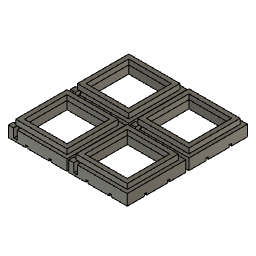
Bitleaf (Autodesk Fusion 360 design; units mm, degrees)
Autodesk Fusion 360 part; units mm, degrees
note: some values were not read from the file. Chosen so that the rebuilt part matches the saved one: which bodies a step acts on; which face or edge a step refers to. Set by a fixed rule: which sketch regions a step uses.
sketch "Skizze1" plane through (0, 0, 0) normal (0, 0, 1) x (1, 0, 0)
  line L0 (0, 0) -> (66.6, 0)
  line L1 (66.6, 0) -> (66.6, -66.6)
  line L2 (66.6, -66.6) -> (0, -66.6)
  line L3 (0, -66.6) -> (0, 0)
  dimension "d1" = 66.6
  dimension "d2" = 66.6
  constraint horizontal L0
  constraint vertical L1
  constraint horizontal L2
  constraint vertical L3
  constraint coincident L0.start L3.end
  measures "d1" distance of L0.start L0.end
  measures "d2" distance of L0.start L2.end
extrude "Extrusion1" add sketch "Skizze1" along normal blind 20 makes body 1
shell "Schale1" thickness 7 outward yes removed faces 1 at (22.2, -22.2, 20) on bodies 1
sketch "Skizze2" plane through (0, 0, 0) normal (0, 0, 1) x (-1, 0, 0)
  line L0 (0, 66.6) -> (-66.6, 66.6)
  line L1 (-66.6, 66.6) -> (-66.6, 0)
  line L2 (-66.6, 0) -> (0, 0)
  line L3 (0, 0) -> (0, 66.6)
  line L4 (0, 0) -> (-66.6, 0)
  line L5 (-66.6, 0) -> (-66.6, 4)
  line L6 (-66.6, 4) -> (0, 4)
  line L7 (0, 4) -> (0, 0)
  line L8 (0, 0) -> (-4, 0)
  line L9 (-4, 0) -> (-4, 66.6)
  line L10 (-4, 66.6) -> (0, 66.6)
  line L11 (0, 66.6) -> (0, 0)
  line L12 (0, 66.6) -> (-66.6, 66.6)
  line L13 (-66.6, 66.6) -> (-66.6, 62.6)
  line L14 (-66.6, 62.6) -> (0, 62.6)
  line L15 (0, 62.6) -> (0, 66.6)
  line L16 (-66.6, 0) -> (-62.6, 0)
  line L17 (-62.6, 0) -> (-62.6, 66.6)
  line L18 (-62.6, 66.6) -> (-66.6, 66.6)
  line L19 (-66.6, 66.6) -> (-66.6, 0)
  dimension "d6" = 66.6
  dimension "d7" = 4
  dimension "d8" = 4
  dimension "d9" = 66.6
  dimension "d10" = 66.6
  dimension "d11" = 4
  dimension "d12" = 4
  dimension "d13" = 66.6
  constraint horizontal L4
  constraint vertical L5
  constraint horizontal L6
  constraint vertical L7
  constraint coincident L2.end L3.start
  constraint horizontal L8
  constraint vertical L9
  constraint horizontal L10
  constraint vertical L11
  constraint horizontal L12
  constraint vertical L13
  constraint horizontal L14
  constraint vertical L15
  constraint coincident L0.start L3.end
  constraint horizontal L16
  constraint vertical L17
  constraint horizontal L18
  constraint vertical L19
  constraint coincident L1.end L2.start
  measures "d6" distance of L2.end L1.end
  measures "d7" distance of L2.end L6.end
  measures "d8" distance of L2.end L8.end
  measures "d9" distance of L2.end L0.start
  measures "d10" distance of L0.start L0.end
  measures "d11" distance of L0.start L14.end
  measures "d12" distance of L1.end L16.end
  measures "d13" distance of L1.end L0.end
extrude "Extrusion2" cut sketch "Skizze2" against normal blind 42 contours L6 L9 L14 L17 bodies 1
sketch "Skizze3" plane through (0, 0, 0) normal (0, 1, 0) x (1, 0, 0)
  line L0 (-7, 7) -> (-2, 7)
  line L1 (-2, 7) -> (-2, 2)
  line L2 (-2, 2) -> (-7, 2)
  line L3 (-7, 2) -> (-7, 7)
  dimension "d16" = 5
  dimension "d17" = 5
  constraint horizontal L0
  constraint vertical L1
  constraint horizontal L2
  constraint vertical L3
  measures "d16" distance of L0.start L0.end
  measures "d17" distance of L0.start L2.end
sketch "Skizze4" plane through (0, -73.6, 0) normal (0, -1, 0) x (1, 0, 0)
  line L0 (-7, -7) -> (73.6, -7)
  line L1 (73.6, -7) -> (73.6, 20)
  line L2 (73.6, 20) -> (-7, 20)
  line L3 (-7, 20) -> (-7, -7)
  line L4 (-7, -7) -> (-2, -7)
  line L5 (-2, -7) -> (-2, -2)
  line L6 (-2, -2) -> (-7, -2)
  line L7 (-7, -2) -> (-7, -7)
  line L8 (73.6, -7) -> (68.6, -7)
  line L9 (68.6, -7) -> (68.6, -2)
  line L10 (68.6, -2) -> (73.6, -2)
  line L11 (73.6, -2) -> (73.6, -7)
  dimension "d18" = 5
  dimension "d19" = 5
  dimension "d20" = 5
  dimension "d21" = 5
  constraint horizontal L4
  constraint vertical L5
  constraint horizontal L6
  constraint vertical L7
  constraint coincident L0.start L3.end
  constraint horizontal L8
  constraint vertical L9
  constraint horizontal L10
  constraint vertical L11
  constraint coincident L0.end L1.start
  measures "d18" distance of L0.start L4.end
  measures "d19" distance of L0.start L6.end
  measures "d20" distance of L0.end L8.end
  measures "d21" distance of L0.end L10.end
extrude "Extrusion3" cut sketch "Skizze4" against normal blind 570 contours L0 L3 L4 L5 L6 L7 bodies 1
sketch "Skizze5" plane through (0, -73.6, 0) normal (0, -1, 0) x (1, 0, 0)
  line L0 (-2, -2) -> (-2, -7)
  line L1 (-2, -7) -> (73.6, -7)
  line L2 (73.6, -7) -> (73.6, 20)
  line L3 (73.6, 20) -> (-7, 20)
  line L4 (-7, 20) -> (-7, -2)
  line L5 (-7, -2) -> (-2, -2)
  line L6 (73.6, -7) -> (68.6, -7)
  line L7 (68.6, -7) -> (68.6, -2)
  line L8 (68.6, -2) -> (73.6, -2)
  line L9 (73.6, -2) -> (73.6, -7)
  dimension "d24" = 5
  dimension "d25" = 5
  constraint horizontal L6
  constraint vertical L7
  constraint horizontal L8
  constraint vertical L9
  constraint coincident L1.end L2.start
  measures "d24" distance of L1.end L6.end
  measures "d25" distance of L1.end L8.end
extrude "Extrusion4" cut sketch "Skizze5" against normal blind 280 contours L1 L2 L6 L7 L8 L9 bodies 1
sketch "Skizze6" plane through (68.6, 0, 0) normal (1, 0, 0) x (0, 1, 0)
  line L0 (7, -7) -> (7, -2)
  line L1 (7, -2) -> (-73.6, -2)
  line L2 (-73.6, -2) -> (-73.6, -7)
  line L3 (-73.6, -7) -> (7, -7)
  line L4 (7, -7) -> (2, -7)
  line L5 (2, -7) -> (2, -2)
  line L6 (2, -2) -> (7, -2)
  line L7 (7, -2) -> (7, -7)
  dimension "d28" = 5
  dimension "d29" = 5
  constraint horizontal L4
  constraint vertical L5
  constraint horizontal L6
  constraint vertical L7
  constraint coincident L0.start L3.end
  measures "d28" distance of L0.start L4.end
  measures "d29" distance of L0.start L0.end
extrude "Extrusion5" cut sketch "Skizze6" against normal blind 135 contours L0 L1 L3 L4 L5 L6 L7 bodies 1
sketch "Skizze7" plane through (68.6, 0, 0) normal (1, 0, 0) x (0, 1, 0)
  line L0 (2, -7) -> (2, -2)
  line L1 (2, -2) -> (-73.6, -2)
  line L2 (-73.6, -2) -> (-73.6, -7)
  line L3 (-73.6, -7) -> (2, -7)
  line L4 (-73.6, -7) -> (-68.6, -7)
  line L5 (-68.6, -7) -> (-68.6, -2)
  line L6 (-68.6, -2) -> (-73.6, -2)
  line L7 (-73.6, -2) -> (-73.6, -7)
  dimension "d32" = 5
  dimension "d33" = 5
  constraint horizontal L4
  constraint vertical L5
  constraint horizontal L6
  constraint vertical L7
  constraint coincident L2.end L3.start
  measures "d32" distance of L2.end L4.end
  measures "d33" distance of L2.end L1.end
extrude "Extrusion6" cut sketch "Skizze7" against normal blind 145 contours L1 L2 L3 L4 L5 L6 L7 bodies 1
sketch "Skizze8" plane through (0, -66.6, 0) normal (0, 1, 0) x (-1, 0, 0)
  line L0 (-66.6, 0) -> (0, 0)
  line L1 (0, 0) -> (0, 20)
  line L2 (0, 20) -> (-66.6, 20)
  line L3 (-66.6, 20) -> (-66.6, 0)
  line L4 (-66.6, 0) -> (-61.6, 0)
  line L5 (-61.6, 0) -> (-61.6, 16)
  line L6 (-61.6, 16) -> (-66.6, 16)
  line L7 (-66.6, 16) -> (-66.6, 0)
  dimension "d36" = 5
  dimension "d37" = 16
  constraint horizontal L4
  constraint vertical L5
  constraint horizontal L6
  constraint vertical L7
  constraint coincident L0.start L3.end
  measures "d36" distance of L0.start L4.end
  measures "d37" distance of L0.start L6.end
extrude "Extrusion7" cut sketch "Skizze8" against normal blind 20 contours L0 L3 L4 L5 L6 L7 bodies 1
sketch "Skizze9" plane through (66.6, 0, 0) normal (-1, 0, 0) x (0, -1, 0)
  line L0 (0, 0) -> (73.6, 0)
  line L1 (73.6, 0) -> (73.6, 16)
  line L2 (73.6, 16) -> (66.6, 16)
  line L3 (66.6, 16) -> (66.6, 20)
  line L4 (66.6, 20) -> (0, 20)
  line L5 (0, 20) -> (0, 0)
  line L6 (66.6, 16) -> (61.6, 16)
  line L7 (61.6, 16) -> (61.6, 0)
  line L8 (61.6, 0) -> (66.6, 0)
  line L9 (66.6, 0) -> (66.6, 16)
  dimension "d40" = 5
  constraint horizontal L6
  constraint vertical L7
  constraint horizontal L8
  constraint vertical L9
  constraint coincident L2.end L3.start
  measures "d40" distance of L2.end L6.end
extrude "Extrusion8" cut sketch "Skizze9" against normal blind 19 contours L0 L6 L7 L8 L9 bodies 1
sketch "Skizze10" plane through (0, 0, 0) normal (0, 0, 1) x (1, 0, 0)
  circle A0 centre (-80, 15) radius 1.5
  line L0 (-78.8067, 15.9088) -> (-74.8067, 15.9088)
  line L1 (-74.8067, 15.9088) -> (-74.8067, 14.0729)
  line L2 (-74.8067, 14.0729) -> (-78.8067, 14.0729)
  line L3 (-78.8067, 14.0729) -> (-78.8067, 15.9088)
  dimension "d43" = 3
  dimension "d44" = 4
  dimension "d45" = 1.836
  constraint horizontal L0
  constraint vertical L1
  constraint horizontal L2
  constraint vertical L3
  constraint coincident A0 L0.start
  measures "d43" diameter of A0
  measures "d44" distance of L0.start L0.end
  measures "d45" distance of L0.start L2.end
sketch "Skizze11" plane through (0, 0, 0) normal (0, 0, 1) x (1, 0, 0)
sketch "Skizze12" plane through (0, 0, 0) normal (0, 0, 1) x (1, 0, 0)
  line L0 (-74.8, 15) -> (-73.607, 15)
  circle A0 centre (-73.607, 15) radius 1.5
  dimension "d46" = 1.193
  dimension "d47" = 3
  constraint horizontal L0
  constraint coincident L0.end A0.centre
  measures "d46" distance of L0.start L0.end
  measures "d47" diameter of A0
extrude "Extrusion9" add sketch "Skizze10" sketch "Skizze12" along normal blind 3 separate body of sketch 2 makes body 2
move_body "Verschieben1" bodies 2 to x (1, 0, 0) y (0, 1, 0) z (0, 0, 1) at (60, -70, 0)
extrude "Extrusion10" add 2 faces at (71.2667, -63.2667, 16) (63.2667, -68.9333, 16) along direction (0, 0, -1) blind 4 on bodies 1 bodies 1
extrude "Extrusion11" cut 1 faces at (44.4, -71.2667, 20) along direction (0, 0, -1) blind 5 on bodies 1 bodies 1
move_body "Verschieben2" bodies 2 to x (1, 0, 0) y (0, 1, 0) z (0, 0, 1) at (9, 0, 17)
move_body "Verschieben3" bodies 2 to x (1, 0, 0) y (0, 1, 0) z (0, 0, 1) at (-2.1624, 3.0539, -2.6132)
sketch "Skizze13" plane through (0, 0, 15) normal (0, 0, 1) x (-1, 0, 0)
  line L0 (0, 66.6) -> (0, 0)
  line L1 (0, 0) -> (-66.6, 0)
  line L2 (-66.6, 0) -> (-66.6, 66.6)
  line L3 (-66.6, 66.6) -> (0, 66.6)
  line L4 (7, 73.6) -> (-73.6, 73.6)
  line L5 (-73.6, 73.6) -> (-73.6, -7)
  line L6 (-73.6, -7) -> (7, -7)
  line L7 (7, -7) -> (7, 73.6)
extrude "Extrusion12" add sketch "Skizze10" sketch "Skizze12" along normal blind 3 separate body of sketch 2 makes body 3
move_body "Verschieben4" bodies 2 to x (1, 0, 0) y (0, 1, 0) z (0, 0, 1) at (-9, 0, 0)
sketch "Skizze14" plane through (0, 0, 15) normal (0, 0, 1) x (-1, 0, 0)
sketch "Skizze15" plane through (0, 0, 0) normal (0, 0, 1) x (1, 0, 0)
  circle A0 centre (-44.5, -48.5) radius 1.8
  circle A1 centre (-50.5, -48.5) radius 1.8
  line L0 (-50.5, -48.5) -> (-44.5, -48.5)
  line L1 (-47.5, -47) -> (-47.5, -50)
  line L2 (-45.0171, -47) -> (-50, -47)
  line L3 (-50, -47) -> (-50, -50)
  line L4 (-50, -50) -> (-45.0171, -50)
  line L5 (-45.0171, -50) -> (-45.0171, -47)
  constraint coincident A1.centre L0.start
  constraint coincident A0.centre L0.end
  constraint horizontal L0
  constraint perpendicular L0 L1
  constraint horizontal L2
  constraint vertical L3
  constraint horizontal L4
  constraint vertical L5
extrude "Extrusion13" add sketch "Skizze15" along normal blind 3 separate body contours A0 L2 L4 L5 | A0 L0 L2 L5 | A0 L0 L1 L2 | A0 L0 L1 L4 | A0 L0 L4 L5 makes body 4
move_body "Verschieben5" bodies 2 to x (1, 0, 0) y (0, 1, 0) z (0, 0, 1) at (-7, 0, 0)
sketch "Skizze16" plane through (0, 0, 15) normal (0, 0, 1) x (-1, 0, 0)
  line L0 (7, 50) -> (-73.6, 50)
  line L1 (7, 50) -> (7, 15)
  line L2 (7, 15) -> (-73.6, 15)
  line L3 (-73.6, 15) -> (-73.6, 50)
  line L4 (-73.6, 73.6) -> (-50, 73.6)
  line L5 (-50, 73.6) -> (-15, 73.6)
  line L6 (-15, 73.6) -> (-15, -7)
  line L7 (-15, -7) -> (-50, -7)
  line L8 (-50, -7) -> (-50, 73.6)
  dimension "d60" = 23.6
  constraint horizontal L0
  constraint perpendicular L0 L1
  constraint perpendicular L1 L2
  constraint perpendicular L0 L3
  constraint horizontal L4
  constraint horizontal L5
  constraint vertical L6
  constraint horizontal L7
  constraint vertical L8
  measures "d60" distance of L4.start L4.end
copy_body "Körper kopieren/einfügen1" bodies 4 makes body 5
move_body "Verschieben6" bodies 5 to x (1, 0, 0) y (0, 1, 0) z (0, 0, 1) at (40.5, 0, 12)
move_body "Verschieben7" bodies 5 to x (1, 0, 0) y (0, 1, 0) z (0, 0, 1) at (-8, 0, 0)
sketch "Skizze17" plane through (0, 0, 0) normal (1, 0, 0) x (0, 1, 0)
sketch "Skizze18" plane through (0, 0, 0) normal (0, 0, 1) x (1, 0, 0)
move_body "Verschieben8" bodies 4 to x (1, 0, 0) y (0, 1, 0) z (0, 0, 1) at (10, 0, 0)
move_body "Verschieben9" bodies 5 to x (1, 0, 0) y (0, 1, 0) z (0, 0, 1) at (8, 0, 0)
split "Teilen1" by bodies 5 bodies 1 makes body 6 at (22.2, -71.2667, 15)
move_body "Verschieben10" bodies 5 to x (1, 0, 0) y (0, 1, 0) z (0, 0, 1) at (0, 32, 0)
split "Teilen2" by bodies 5 bodies 6 makes body 7 at (22.2, -71.2667, 15)
move_body "Verschieben11" bodies 5 to x (0, -1, 0) y (1, 0, 0) z (0, 0, 1) at (33, 0, 0)
split "Teilen3" by bodies 5 bodies 7 makes body 8 at (44.4, -71.2667, 15)
move_body "Verschieben12" bodies 5 to x (1, 0, 0) y (0, 1, 0) z (0, 0, 1) at (32, 0, 0)
split "Teilen4" by bodies 5 bodies 8 makes body 9 at (44.4, -71.2667, 15)
move_body "Verschieben13" bodies 5 to x (0, -1, 0) y (1, 0, 0) z (0, 0, 1) at (66.6, 32, 0)
split "Teilen5" by bodies 5 bodies 9 makes body 10 at (44.4, -71.2667, 15)
move_body "Verschieben14" bodies 5 to x (1, 0, 0) y (0, 1, 0) z (0, 0, 1) at (0, -32, 0)
split "Teilen6" by bodies 5 bodies 10 makes body 11 at (22.2, -71.2667, 15)
move_body "Verschieben15" bodies 5 to x (0, -1, 0) y (1, 0, 0) z (0, 0, 1) at (97, 0, 0)
split "Teilen7" by bodies 5 bodies 11 makes body 12 at (13.3333, -71.2667, 15)
move_body "Verschieben16" bodies 5 to x (1, 0, 0) y (0, 1, 0) z (0, 0, 1) at (-32, 0, 0)
split "Teilen8" by bodies 5 bodies 12 makes body 13 at (71.2667, -63.4, 15)
move_body "Verschieben17" bodies 5 to x (1, 0, 0) y (0, 1, 0) z (0, 0, 1) at (0, -30, 0)
move_body "Verschieben18" bodies 2 to x (1, 0, 0) y (0, 1, 0) z (0, 0, 1) at (55, 0, 0)
extrude "Extrusion14" cut 1 faces at (28.3642, -51.0373, 15.3868) along direction (0, -1, 0) blind 0.1 on bodies 2 bodies 2
extrude "Extrusion15" cut 1 faces at (29.6976, -52.8732, 15.3868) along direction (0, 1, 0) blind 0.1 on bodies 2 bodies 2
sketch "Skizze19" plane through (0, 0, 14.3868) normal (0, 0, -1) x (1, 0, 0)
  line L0 (31.0309, 52.8465) -> (31.0309, 52.7732)
  line L1 (31.0309, 52.7732) -> (27.0309, 52.7732)
  line L2 (27.0309, 52.7732) -> (27.0309, 52.8549)
  arc A0 (27.0309, 52.8549) -> (27.0309, 51.0373) centre (25.8376, 51.9461) ccw
  line L3 (27.0309, 51.0373) -> (27.0309, 51.1373)
  line L4 (27.0309, 51.1373) -> (31.0309, 51.1373)
  line L5 (31.0309, 51.1373) -> (31.0309, 51.0457)
  arc A1 (31.0309, 51.0457) -> (31.0309, 52.8465) centre (32.2306, 51.9461) ccw
  circle A2 centre (25.8376, 51.9461) radius 1.45
  circle A3 centre (32.2306, 51.9461) radius 1.45
  dimension "d65" = 2.9
  dimension "d66" = 2.9
  constraint concentric A0 A2
  constraint concentric A1 A3
  measures "d65" diameter of A2
  measures "d66" diameter of A3
extrude "Extrusion16" add sketch "Skizze15" along normal blind 3 separate body makes body 14
extrude "Extrusion17" cut 2 faces at (-48.1683, -47, 2) (-46.1633, -47, 1) along direction (0, -1, 0) blind 0.25 on bodies 14 bodies 14
extrude "Extrusion18" cut 1 faces at (-48.1683, -50, 1) along direction (0, 1, 0) blind 0.25 on bodies 14 bodies 14
move_body "Verschieben19" bodies 14 to x (1, 0, 0) y (0, 1, 0) z (0, 0, 1) at (85, 0, 0)
move_body "Verschieben20" bodies 14 13 to x (-1, 0, 0) y (0, 1, 0) z (0, 0, -1) at (123.2, 0, 12)
move_body "Verschieben21" bodies 14 to x (1, 0, 0) y (0, 1, 0) z (0, 0, 1) at (0, 0, -10)
extrude "Extrusion19" cut 1 faces at (128.5333, -21.5333, 14) along direction (0, 0, -1) blind 2 on bodies 13 bodies 13
copy_body "Körper kopieren/einfügen2" bodies 13 makes body 15
move_body "Verschieben22" bodies 15 to x (1, 0, 0) y (0, 1, 0) z (0, 0, 1) at (83, 0, 0)
copy_body "Körper kopieren/einfügen3" bodies 15 13 makes body 16 makes body 17
move_body "Verschieben23" bodies 16 17 to x (1, 0, 0) y (0, 1, 0) z (0, 0, 1) at (0, -85, 0)
hidden bodies 1 2 3 4 5 6 7 8 9 10 11 12
named bodies: "Bauteil", "Knochen", "Verbindung", "Verbindung (1)", "Bauteil (1)", "Bauteil (1) (1)", "Bauteil (1) (1) (1)", "Bauteil (1) (1) (1) (1)", "Bauteil (1) (1) (1) (1) (1)", "Bauteil (1) (1) (1) (1) (1) (1)", "Bauteil (1) (1) (1) (1) (1) (1) (1)", "Bauteil (1) (1) (1) (1) (1) (1) (1) (1)", "true connection", "Bauteil (1) (1) (1) (1) (1) (1) (1) (1) (1)", "Bauteil (1) (1) (1) (1) (1) (1) (1) (1) (2)", "Bauteil (1) (1) (1) (1) (1) (1) (1) (1) (1) (1)"
